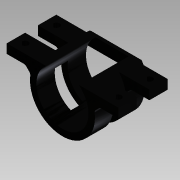
# Autodesk Inventor part: DudukanKipas
Saved by Autodesk Inventor 2015 SP1 (Build 190203100, 203)
## iProperties
Created: 2015-02-01
Part Number: DudukanKipas
Material: Generic
Document SubType Name: Modeling
Designer: Rafi Kurnia Putra
Density: 1 g/cm^3
Appearance: Smooth - Purple
Mass: 12.1783 g
Surface Area: 74.2447 cm^2
Volume: 12.1783 cm^3
Author: Rafi Kurnia Putra
Autodesk Inventor part; units mm, degrees
ref_plane "YZ Plane" through (0, 0, 0) normal (1, 0, 0) x (0, 1, 0)
ref_plane "XZ Plane" through (0, 0, 0) normal (0, 1, 0) x (-1, 0, 0)
ref_plane "XY Plane" through (0, 0, 0) normal (0, 0, 1) x (1, 0, 0)
sketch "Sketch1" plane through (0, 0, 0) normal (0, 1, 0) x (-1, 0, 0)
  arc A0 (-17.5649, 2.183) -> (17.5649, 2.183) centre (0, 0) ccw
  line L0 (-21.1184, 5.9985) -> (-30.35, 5.9985)
  line L1 (30.35, 5.9985) -> (30.35, 10.9985)
  line L2 (-30.35, 5.9985) -> (-30.35, 10.9985)
  line L3 (19.7042, 5.4127) -> (18.1354, 3.8439)
  line L4 (21.1184, 5.9985) -> (23.3371, 5.9985) construction
  line L5 (-19.7042, 5.4127) -> (-18.1354, 3.8439)
  line L6 (-16.6526, 5.9985) -> (-16.2328, 5.9985) construction
  arc A1 (18.1354, 3.8439) -> (17.5649, 2.183) centre (19.5496, 2.4297) ccw
  arc A2 (-17.5649, 2.183) -> (-18.1354, 3.8439) centre (-19.5496, 2.4297) ccw
  arc A3 (21.1184, 5.9985) -> (19.7042, 5.4127) centre (21.1184, 3.9985) ccw
  arc A4 (-19.7042, 5.4127) -> (-21.1184, 5.9985) centre (-21.1184, 3.9985) ccw
  arc A5 (-6.35, 10.9985) -> (6.35, 10.9985) centre (0, 0) ccw
  line L7 (30.35, 10.9985) -> (6.35, 10.9985)
  line L8 (-6.35, 10.9985) -> (-30.35, 10.9985)
  line L9 (30.35, 5.9985) -> (21.1184, 5.9985)
  point P0 (17.4211, 3.1296)
  point P1 (-17.4211, 3.1296)
  dimension "d9" = 135
  dimension "d10" = 45
  dimension "d21" = 2
  dimension "d22" = 25.4
  dimension "d55" = 5
  constraints: 20 end point, 15 point on circle, 8 tangent, 6 centre point, 3 equal radius, 3 horizontal, 2 coincident, 2 point on line, 1 collinear, 1 equal length, 1 parallel, 1 perpendicular, 1 vertical
  measures "d9" angle of L3 L4
  measures "d10" angle of L5 L6
  measures "d21" radius of A1
  measures "d22" diameter of A5
  measures "d55" distance of L0.end L2.end
extrude "Extrusion1" add sketch "Sketch1" along normal blind 10
sketch "Sketch2" plane through (-30.35, 0, 10.9985) normal (0, 0, 1) x (1, 0, 0)
  circle A0 centre (5, 5) radius 1.75
  circle A1 centre (55.7001, 5) radius 1.75
  line L0 (0, 0) -> (0, 10) projected
  line L1 (60.7001, 0) -> (60.7001, 10) projected
  line L2 (36.7001, 0) -> (36.7001, 10) projected
  line L3 (24, 0) -> (24, 10) projected
  point P0 (30.35, 0)
  dimension "d25" = 3.5
  dimension "d26" = 3.5
  dimension "d27" = 5
  dimension "d28" = 5
  dimension "d30" = 12.7001
  constraints: 2 centre point
  measures "d25" diameter of A0
  measures "d26" diameter of A1
  measures "d27" distance from line of L0 A0.centre
  measures "d28" distance from line of L1 A1.centre
  measures "d30" distance between parallel lines of L2 L3
extrude "Extrusion2" cut sketch "Sketch2" against normal through all
sketch "Sketch3" plane through (0, 0, 0) normal (0, -1, 0) x (1, 0, 0)
  line L0 (13.8681, 10.9985) -> (6.35, 10.9985)
  line L1 (-12.5071, 2.2053) -> (-17.4311, 3.0736)
  line L2 (12.5071, 2.2053) -> (17.4311, 3.0736)
  arc A0 (-6.35, 10.9985) -> (-12.5071, 2.2053) centre (0, 0) ccw
  arc A1 (12.5071, 2.2053) -> (6.35, 10.9985) centre (0, 0) ccw
  line L3 (-4.8601, -11.7333) -> (-6.7735, -16.3527)
  line L4 (4.8601, -11.7333) -> (6.7735, -16.3527)
  line L5 (-6.35, 10.9985) -> (-13.8681, 10.9985)
  line L6 (13.8681, 10.9985) -> (6.35, 10.9985)
  arc A2 (-6.35, 10.9985) -> (-12.5071, 2.2053) centre (0, 0) ccw
  arc A3 (-13.8681, 10.9985) -> (-17.4311, 3.0736) centre (0, 0) ccw
  arc A4 (-4.8601, -11.7333) -> (4.8601, -11.7333) centre (0, 0) ccw
  arc A5 (12.5071, 2.2053) -> (6.35, 10.9985) centre (0, 0) ccw
  arc A6 (-6.7735, -16.3527) -> (6.7735, -16.3527) centre (0, 0) ccw
  arc A7 (17.4311, 3.0736) -> (13.8681, 10.9985) centre (0, 0) ccw
  arc A8 (17.4311, 3.0736) -> (13.8681, 10.9985) centre (0, 0) ccw
  arc A9 (-13.8681, 10.9985) -> (-17.4311, 3.0736) centre (0, 0) ccw
  arc A10 (-6.7735, -16.3527) -> (6.7735, -16.3527) centre (0, 0) ccw
  constraints: 22 point on circle, 14 end point, 11 centre point
extrude "Extrusion3" add sketch "Sketch3" along normal blind 3.5
mirror "Mirror2" about plane through (12.3952, -3.5, 7.3622) normal (0, -1, 0) of "Extrusion1", "Extrusion3"
sketch "Sketch13" plane through (-30.35, 10, 10.9985) normal (0, 0, 1) x (1, 0, 0)
  circle A0 centre (5, -5) radius 1.75 projected
  line L0 (0, -10) -> (0, 0) projected
  line L1 (0, 0) -> (24, 0) projected
  circle A1 centre (5, -22) radius 1.75
  circle A2 centre (55.7001, -22) radius 1.75
  line L2 (0, -27) -> (24, -27) projected
  circle A3 centre (55.7001, -5) radius 1.75 projected
  point P0 (30.35, -10)
  dimension "d60" = 5
  dimension "d61" = 5
  dimension "d62" = 3.5
  dimension "d63" = 3.5
  dimension "d64" = 5
  constraints: 2 centre point, 1 horizontal alignment, 1 vertical alignment
  measures "d60" distance from line of L0 A0.centre
  measures "d61" distance from line of A0.centre L1
  measures "d62" diameter of A1
  measures "d63" diameter of A2
  measures "d64" distance from line of L2 A1.centre
extrude "Extrusion7" cut sketch "Sketch13" against normal through all contours A1 | A2
sketch "Sketch14" plane through (0, 10, 0) normal (0, 1, 0) x (1, 0, 0)
  arc A0 (-17.4311, -3.0736) -> (-13.8681, -10.9985) centre (0, 0) ccw
  arc A1 (13.8681, -10.9985) -> (17.4311, -3.0736) centre (0, 0) ccw
  line L0 (-13.8681, -10.9985) -> (13.8681, -10.9985)
  line L1 (17.4311, -3.0736) -> (-17.4311, -3.0736)
  constraints: 4 end point, 4 point on circle, 2 centre point, 1 horizontal, 1 parallel
extrude "Extrusion8" add sketch "Sketch14" along normal blind 3
fillet "Fillet1" radius 2 4 edges at (16.1434, 13, 7.2581) (-16.1434, 13, 7.2581) (0, 13, 3.0736) (0, 13, 10.9985)
sketch "Sketch15" plane through (0, -17, 0) normal (0, -1, 0) x (1, 0, 0)
  arc A0 (-6.35, 10.9985) -> (6.35, 10.9985) centre (0, 0) ccw projected
  arc A1 (-12.3225, 3.0736) -> (12.3225, 3.0736) centre (0, 0) ccw projected
  circle A2 centre (0, 0) radius 12.7
  circle A3 centre (0, 0) radius 14.2
  dimension "d71" = 1.5
  constraints: 2 centre point, 1 coincident, 1 other
  measures "d71" radial gap between concentric circles of A3 A2
extrude "Extrusion9" cut sketch "Sketch15" against normal blind 27
sketch "Sketch18" plane through (0, 13, 0) normal (0, 1, 0) x (1, 0, 0)
  arc A0 (-13.8634, -3.0736) -> (-13.2385, -5.0736) centre (-0.5126, 0) ccw
  arc A1 (13, -5.0736) -> (13.8634, -3.0736) centre (7.2228, -1.3933) ccw
  line L0 (-13.2385, -5.0736) -> (13, -5.0736)
  line L1 (13.8634, -3.0736) -> (-13.8634, -3.0736)
  point P0 (0, 0)
  constraints: 4 end point, 4 point on circle, 2 centre point, 1 horizontal
extrude "Extrusion10" cut sketch "Sketch18" against normal through all
sketch "Sketch19" plane through (0, 0, 0) normal (1, 0, 0) x (0, 1, 0)
  spline S0 degree 6 poles (11, 3.0736) (11.2241, 3.0736) (11.4486, 3.1037) (11.6701, 3.1642) (11.8849, 3.2555) (12.0884, 3.3783) (12.3206, 3.5704) (12.3653, 3.6101) (12.4088, 3.6516) (12.451, 3.6949) (12.4917, 3.74) (12.5992, 3.8679) (12.663, 3.9542) (12.7214, 4.0451) (12.7739, 4.1397) (12.82, 4.2374) (12.9073, 4.4579) (12.9453, 4.5813) (12.9733, 4.706) (12.9914, 4.8306) (13, 4.9536) (13, 5.0736) knots 0 0 0 0 0 0 0 0.457146 0.457146 0.457146 0.457146 0.457146 0.569315 0.569315 0.569315 0.569315 0.569315 0.764458 0.764458 0.764458 0.764458 0.764458 1 1 1 1 1 1 1 projected
  line L0 (10, 3.0736) -> (11, 3.0736) projected
  line L1 (10, 5.0736) -> (10, 3.0736) projected
  line L2 (13, 5.0736) -> (10, 5.0736) projected
  point P0 (0, 0)
  constraints: 1 other
extrude "Extrusion11" cut sketch "Sketch19" along normal mid plane 200
body "Solid1"
